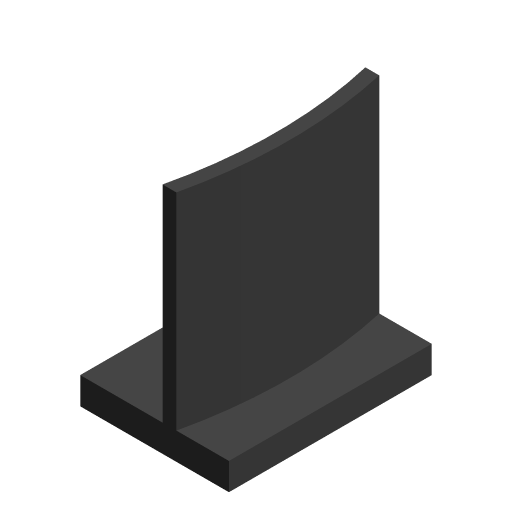
# Autodesk Inventor part: Camera retention
Saved by Autodesk Inventor 2024 (Build 280153000, 153)
## iProperties
Part Number: Camera retention
Material: Generic
Document SubType Name: Modeling
Designer: Jamie
Appearance: Default
Author: Jamie
Autodesk Inventor part; units mm, degrees
ref_plane "YZ Plane" through (0, 0, 0) normal (1, 0, 0) x (0, 1, 0)
ref_plane "XZ Plane" through (0, 0, 0) normal (0, 1, 0) x (-1, 0, 0)
ref_plane "XY Plane" through (0, 0, 0) normal (0, 0, 1) x (1, 0, 0)
sketch "Sketch3" plane through (0, 0, 0) normal (0, 1, 0) x (-1, 0, 0)
  circle A0 centre (0, 0) radius 33
  circle A1 centre (0, 0) radius 34
  line L0 (-30.4296, 7.5) -> (-38.9548, 7.5)
  line L1 (-38.9548, 7.5) -> (-38.9548, -7.5)
  line L2 (-38.9548, -7.5) -> (-30.4296, -7.5)
  line L3 (-30.4296, -7.5) -> (-30.4296, 7.5)
  point P0 (-33.1625, -7.5)
  point P1 (-32.1364, -7.5)
  point P2 (-32.1364, 7.5)
  point P3 (-33.1625, 7.5)
  dimension "d9" = 66
  dimension "d10" = 68
  dimension "d11" = 7.5
  dimension "d12" = 7.5
  constraints: 8 end point, 2 centre point, 2 coincident, 2 parallel, 1 horizontal, 1 perpendicular
  measures "d9" diameter of A0
  measures "d10" diameter of A1
  measures "d11" distance from line of point (0, 0) L0
  measures "d12" distance from line of point (0, 0) L2
extrude "Extrusion2" add sketch "Sketch3" along normal blind 15.25 contours A0 L2 A1 L0 picked at (-32.7342, -5.8399)
sketch "Sketch4" plane through (0, 0, 0) normal (0, -1, 0) x (1, 0, 0)
  line L0 (26.0495, 7.5) -> (37.0495, 7.5)
  line L1 (37.0495, 7.5) -> (37.0495, -7.5)
  line L2 (37.0495, -7.5) -> (26.0495, -7.5)
  line L3 (26.0495, -7.5) -> (26.0495, 7.5)
  line L4 (33.1625, -7.5) -> (32.1364, -7.5) projected
  line L5 (32.1364, 7.5) -> (33.1625, 7.5) projected
  point P0 (0, 0)
  point P1 (32.6495, -7.5)
  point P2 (32.6495, -7.5)
  dimension "d15" = 6.6
  dimension "d16" = 4.4
  dimension "d17" = 0
  dimension "d18" = 0
  constraints: 8 end point, 2 midpoint, 2 parallel, 1 horizontal, 1 perpendicular
  measures "d15" distance from line of L3 point (32.649, -7.5)
  measures "d16" distance from line of point (32.649, -7.5) L1
  measures "d17" distance between parallel lines of L4 L2
  measures "d18" distance between parallel lines of L5 L0
extrude "Extrusion3" add sketch "Sketch4" along normal blind 2
sketch "Sketch5" plane through (0, -2, 0) normal (0, -1, 0) x (1, 0, 0)
  circle A0 centre (29.0005, 0) radius 2
  line L0 (37.0495, 7.5) -> (26.0495, 7.5) projected
  line L1 (32.1364, 7.5) -> (33.1625, 7.5) projected
  point P0 (0, 0)
  point P1 (32.6495, 7.5)
  dimension "d21" = 4
  dimension "d22" = 7.5
  dimension "d23" = 3.649
  constraints: 1 centre point, 1 midpoint
  measures "d21" diameter of A0
  measures "d22" distance from line of L0 A0.centre
  measures "d23" horizontal distance of point (32.649, 7.5) A0.centre
extrude "Extrusion4" cut sketch "Sketch5" against normal blind 2
body "Solid2"
